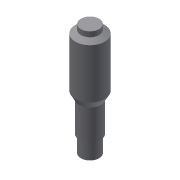
# Autodesk Inventor part: 00_RS_Pro_Micrometer_small
Saved by Autodesk Inventor 2019.4 (Build 234330000, 330)
## iProperties
Created: 2021-10-17
Part Number: 00_RS_Pro_Micrometer_small
Material: Generic
Document SubType Name: Modeling
Designer: diederichbenedict
Density: 1 g/cm^3
Appearance: Default
Author: diederichbenedict
Autodesk Inventor part; units mm, degrees
ref_plane "YZ Plane" through (0, 0, 0) normal (1, 0, 0) x (0, 1, 0)
ref_plane "XZ Plane" through (0, 0, 0) normal (0, 1, 0) x (-1, 0, 0)
ref_plane "XY Plane" through (0, 0, 0) normal (0, 0, 1) x (1, 0, 0)
sketch "Sketch1" plane through (0, 0, 0) normal (1, 0, 0) x (0, 1, 0)
  line L0 (0, 0) -> (0, -1.725)
  line L1 (0, -1.725) -> (0.86, -1.725)
  line L2 (0.86, -1.725) -> (0.86, -3.005)
  line L3 (0.86, -3.005) -> (6.36, -3.005)
  line L4 (6.36, -3.005) -> (6.36, -3.505)
  line L5 (6.36, -3.505) -> (16.28, -3.505)
  line L6 (16.28, -3.505) -> (18.6408, -4.815)
  line L7 (18.6408, -4.815) -> (34.9681, -4.815)
  line L8 (34.9681, -4.815) -> (35.9725, -3.005)
  line L9 (35.9725, -3.005) -> (37.64, -3.005)
  line L10 (37.64, -3.005) -> (37.64, 0)
  line L11 (37.64, 0) -> (0, 0)
  dimension "d0" = 1.725
  dimension "d1" = 0.86
  dimension "d2" = 1.28
  dimension "d3" = 90
  dimension "d4" = 5.5
  dimension "d5" = 0.5
  dimension "d6" = 9.92
  dimension "d7" = 4.815
  dimension "d8" = 37.64
  constraints: 24 end point, 7 perpendicular, 3 point on line, 2 parallel, 1 vertical
  measures "d0" distance of L0.start L0.end
  measures "d1" distance of L0.end L1.end
  measures "d2" distance of L1.end L2.end
  measures "d3" angle of L1 L2
  measures "d4" distance of L2.end L3.end
  measures "d5" distance of L3.end L4.end
  measures "d6" distance of L4.end L5.end
  measures "d7" distance between parallel lines of L11 L7
  measures "d8" distance between parallel lines of L0 L10
revolve "Revolution1" add sketch "Sketch1" angle 360 about axis through (0, 37.64, 0) along (0, -1, 0)
body "Solid1"
